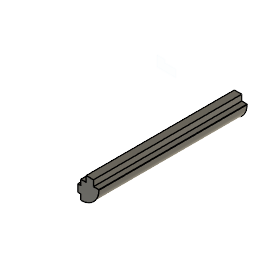
STOP LIGHT FINAL (Autodesk Fusion 360 archive; units mm, degrees)
design "FINAL STOP LIGHT CONNECTOR"
Autodesk Fusion 360 part; units mm, degrees
sketch "Sketch1" plane through (0, 0, 52.25) normal (0, 0, 1) x (-1, 0, 0)
  line L0 (12.25, -100) -> (12.25, 0)
  line L1 (12.25, 0) -> (0, 0)
  line L2 (0, 0) -> (0, -100)
  line L3 (0, -100) -> (12.25, -100)
  line L4 (0, 0) -> (12.25, 0) construction
  line L5 (6.125, 0) -> (8.625, 0) construction
  line L6 (6.125, 0) -> (3.625, 0) construction
  line L7 (3.625, 0) -> (8.625, 0) construction
  line L8 (3.625, 0) -> (8.625, 0)
  line L9 (8.625, 0) -> (8.625, -100)
  line L10 (8.625, -100) -> (3.625, -100)
  line L11 (3.625, -100) -> (3.625, 0)
  dimension "d3" = 5
  constraint coincident L1.end L2.start
  constraint coincident L0.end L1.start
  constraint midpoint L4 L5.start
  constraint horizontal L8
  constraint vertical L9
  constraint horizontal L10
  constraint vertical L11
  constraint coincident L3 L9.end
  measures "d3" distance of L6.end L5.end
sketch "Sketch2" plane through (0, 100, 0) normal (0, 1, 0) x (-1, 0, 0)
  line L0 (-4, 8.6) -> (-4, 3.6)
  line L1 (-4, 3.6) -> (8.5, 3.6)
  line L2 (8.5, 3.6) -> (8.5, 10.6)
  line L3 (8.5, 10.6) -> (3.5, 10.6)
  line L4 (3.5, 10.6) -> (3.5, 8.6)
  line L5 (3.5, 8.6) -> (-4, 8.6)
sketch "Sketch3" plane through (0, 100, 0) normal (0, 1, 0) x (-1, 0, 0)
  line L0 (-43.625, 52.25) -> (-43.625, 50.25)
  line L1 (-43.625, 50.25) -> (-48.625, 50.25)
  line L2 (-48.625, 50.25) -> (-48.625, 52.25)
  line L3 (-48.625, 52.25) -> (-52.25, 52.25)
  line L4 (-52.25, 52.25) -> (-52.25, 12.25)
  line L5 (-52.25, 12.25) -> (-48.625, 12.25)
  line L6 (-48.625, 12.25) -> (-48.625, 16.25)
  line L7 (-48.625, 16.25) -> (-43.625, 16.25)
  line L8 (-43.625, 16.25) -> (-43.625, 12.25)
  line L9 (-43.625, 12.25) -> (-40, 12.25)
  line L10 (-40, 12.25) -> (-40, 52.25)
  line L11 (-40, 52.25) -> (-43.625, 52.25)
  line L12 (-40, 0) -> (-56, 0) construction
  line L13 (-52.25, 12.25) -> (-48.625, 12.25)
  line L14 (-48.625, 16.25) -> (-48.625, 12.25)
  line L15 (-43.625, 16.25) -> (-48.625, 16.25)
  line L16 (-43.625, 12.25) -> (-43.625, 16.25)
  line L17 (-40, 12.25) -> (-43.625, 12.25)
  line L18 (-40, 8.6) -> (-40, 12.25)
  line L19 (-38, 8.6) -> (-40, 8.6)
  line L20 (-38, 3.6) -> (-38, 8.6)
  line L21 (-40, 3.6) -> (-38, 3.6)
  line L22 (-40, 0) -> (-40, 3.6)
  line L23 (-40, 0) -> (-52.25, 0)
  line L24 (-52.25, 12.25) -> (-52.25, 0)
  constraint coincident L4.end L5.start
  constraint horizontal L12
  constraint coincident L5.end L6.start
  constraint coincident L6.end L7.start
  constraint coincident L7.end L8.start
  constraint coincident L8.end L9.start
  constraint coincident L9.end L10.start
  constraint horizontal L19
  constraint perpendicular L19 L20
  constraint perpendicular L20 L21
  constraint coincident L12 L23.end
extrude "Extrude3" add sketch "Sketch3" against normal blind 100 contours L5 L6 L7 L8 L9 L13 L14 L15 L16 L17 L18 L19 L20 L21 L22 L23 L24
fillet "Fillet1" radius 12 1 edges at (52.25, 50, 0)

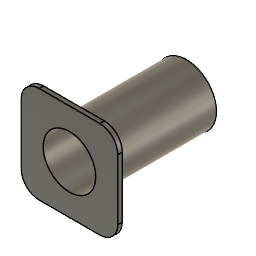
design "connector to base plate"
Autodesk Fusion 360 part; units mm, degrees
sketch "Sketch1" plane through (0, 0, 52.25) normal (0, 0, 1) x (-1, 0, 0)
  line L0 (12.25, -100) -> (12.25, 0)
  line L1 (12.25, 0) -> (0, 0)
  line L2 (0, 0) -> (0, -100)
  line L3 (0, -100) -> (12.25, -100)
  line L4 (0, 0) -> (12.25, 0) construction
  line L5 (6.125, 0) -> (8.625, 0) construction
  line L6 (6.125, 0) -> (3.625, 0) construction
  line L7 (3.625, 0) -> (8.625, 0) construction
  line L8 (3.625, 0) -> (8.625, 0)
  line L9 (8.625, 0) -> (8.625, -100)
  line L10 (8.625, -100) -> (3.625, -100)
  line L11 (3.625, -100) -> (3.625, 0)
  dimension "d3" = 5
  constraint coincident L1.end L2.start
  constraint coincident L0.end L1.start
  constraint midpoint L4 L5.start
  constraint horizontal L8
  constraint vertical L9
  constraint horizontal L10
  constraint vertical L11
  constraint coincident L3 L9.end
  measures "d3" distance of L6.end L5.end
extrude "Extrude1" add sketch "Sketch1" along normal blind 5 contours L1 L3 L8 L9 L10 L11
extrude "Extrude2" cut 1 faces at (-5.2917, 66.6667, 57.25) along direction (0, 0, -1) blind 10
sketch "Sketch2" plane through (0, 100, 0) normal (0, 1, 0) x (-1, 0, 0)
  line L0 (-4, 8.6) -> (-4, 3.6)
  line L1 (-4, 3.6) -> (8.5, 3.6)
  line L2 (8.5, 3.6) -> (8.5, 10.6)
  line L3 (8.5, 10.6) -> (3.5, 10.6)
  line L4 (3.5, 10.6) -> (3.5, 8.6)
  line L5 (3.5, 8.6) -> (-4, 8.6)
sketch "Sketch3" plane through (52.1964, 100, 12.1825) normal (0, 1, 0) x (0, 0, -1)
  line L0 (12.1825, 12.1964) -> (8.5825, 12.1964)
  line L1 (8.5825, 12.1964) -> (8.5825, 14.1964)
  line L2 (8.5825, 14.1964) -> (3.5825, 14.1964)
  line L3 (3.5825, 14.1964) -> (3.5825, 12.1964)
  line L4 (3.5825, 12.1964) -> (-0.0675, 12.1964)
  line L5 (-0.0675, 12.1964) -> (-0.0675, 8.5714)
  line L6 (-0.0675, 8.5714) -> (-4.0675, 8.5714)
  line L7 (-4.0675, 8.5714) -> (-4.0675, 3.5714)
  line L8 (-4.0675, 3.5714) -> (-0.0675, 3.5714)
  line L9 (-0.0675, 3.5714) -> (-0.0675, -0.0536)
  line L10 (-0.0675, -0.0536) -> (0.1825, -0.0536)
  line L11 (12.1825, 11.9464) -> (12.1825, 12.1964)
  line L12 (12.1825, 11.9464) -> (-52.2495, 11.9464)
  line L13 (-52.2495, 11.9464) -> (-52.2495, 76.3784)
  line L14 (-52.2495, 76.3784) -> (12.1825, 76.3784)
  line L15 (12.1825, 76.3784) -> (12.1825, 11.9464)
  arc A0 (0.1825, -0.0536) -> (12.1825, 11.9464) centre (0.1825, 11.9464) ccw
  dimension "d8" = 64.432
  dimension "d9" = 64.432
  constraint vertical L13
  constraint perpendicular L12 L13
  constraint horizontal L14
  constraint parallel L13 L15
  constraint coincident L11.start L12.start
  measures "d8" distance of L11.start L12.end
  measures "d9" distance of L11.start L14.end
extrude "Extrude3" add sketch "Sketch3" along normal blind 3 contours L0 L1 L2 L3 L4 L5 L11 L12 L15 | L0 L1 L2 L3 L4 L5 L12 L13 L14 L15
sketch "Sketch4" plane through (0, 103, 0) normal (0, 1, 0) x (-1, 0, 0)
  line L0 (24.182, 0) -> (24.182, 64.432)
  line L1 (24.182, 64.432) -> (-40.25, 64.432)
  line L2 (-40.25, 64.432) -> (-40.25, 0)
  line L3 (-40.25, 0) -> (24.182, 0)
  line L4 (24.182, 64.432) -> (-40.25, 0) construction
  line L5 (24.182, 0) -> (-40.25, 64.432) construction
  circle A0 centre (-8.034, 32.216) radius 17.5
  circle A1 centre (-8.034, 32.216) radius 20
  dimension "d12" = 35
  dimension "d13" = 40
  constraint coincident L0.end L1.start
  constraint coincident L2.end L3.start
  constraint coincident L0.start L3.end
  constraint coincident L1.end L2.start
  constraint midpoint L5 A0.centre
  constraint concentric A0 A1
  measures "d12" diameter of A0
  measures "d13" diameter of A1
extrude "Extrude4" add sketch "Sketch4" along normal blind 75 contours A1
extrude "Extrude5" cut 1 faces at (9.2669, 103, 37.0337) along direction (0, -1, 0) blind 16
move_body "Move1" bodies 1 to x (1, 0, 0) y (0, 1, 0) z (0, 0, 1) at (0, 0, -12)
sketch "Sketch5" plane through (0, 103, 0) normal (0, 1, 0) x (-1, 0, 0)
  line L0 (-40.25, -12) -> (24.182, -12)
  line L1 (24.182, -12) -> (24.182, 52.432)
  line L2 (24.182, 52.432) -> (-40.25, 52.432)
  line L3 (-40.25, 52.432) -> (-40.25, -12)
  circle A0 centre (-8.034, 20.216) radius 20
fillet "Fillet1" radius 12 4 edges at (40.25, 101.5, -12) (40.25, 101.5, 52.432) (-24.182, 101.5, 52.432) (-24.182, 101.5, -12)

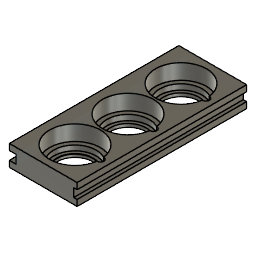
design "stop light"
Autodesk Fusion 360 part; units mm, degrees
sketch "Sketch1" plane through (0, 0, 0) normal (0, 0, 1) x (1, 0, 0)
  line L0 (0, 0) -> (40, 0)
  line L1 (40, 0) -> (40, 100)
  line L2 (40, 100) -> (0, 100)
  line L3 (0, 100) -> (0, 0)
  circle A0 centre (20, 50) radius 12.5
  circle A1 centre (20, 81.25) radius 12.5
  line L4 (5, 81.25, 3.25) -> (5, 66.25, 3.25)
  line L5 (5, 66.25, 3.25) -> (20, 66.25, 3.25)
  line L6 (35, 81.25, 3.25) -> (35, 96.25, 3.25)
  line L7 (35, 96.25, 3.25) -> (20, 96.25, 3.25)
  line L8 (35, 96.25, 3.25) -> (5, 96.25, 3.25)
  line L9 (5, 96.25, 3.25) -> (5, 66.25, 3.25)
  line L10 (5, 66.25, 3.25) -> (35, 66.25, 3.25)
  line L11 (35, 66.25, 3.25) -> (35, 96.25, 3.25)
  line L12 (5, 50, 3.25) -> (5, 65, 3.25)
  line L13 (5, 65, 3.25) -> (20, 65, 3.25)
  line L14 (35, 50, 3.25) -> (35, 35, 3.25)
  line L15 (35, 35, 3.25) -> (20, 35, 3.25)
  line L16 (35, 35, 3.25) -> (5, 35, 3.25)
  line L17 (5, 35, 3.25) -> (5, 65, 3.25)
  line L18 (5, 65, 3.25) -> (35, 65, 3.25)
  line L19 (35, 65, 3.25) -> (35, 35, 3.25)
  line L20 (5, 18.75, 3.25) -> (5, 3.75, 3.25)
  line L21 (5, 3.75, 3.25) -> (20, 3.75, 3.25)
  line L22 (35, 18.75, 3.25) -> (35, 33.75, 3.25)
  line L23 (35, 33.75, 3.25) -> (19.9836, 33.75, 3.25)
  line L24 (35, 33.75, 3.25) -> (5, 33.75, 3.25)
  line L25 (5, 33.75, 3.25) -> (5, 3.75, 3.25)
  line L26 (5, 3.75, 3.25) -> (35, 3.75, 3.25)
  line L27 (35, 3.75, 3.25) -> (35, 33.75, 3.25)
  circle A2 through (32.4836, 18.7208, 0.25) (13.7336, 29.5461, 0.25) (13.7336, 7.8955, 0.25)
  line L28 (5, 96.25, 3.25) -> (5, 100, 3.25) construction
  dimension "d1" = 40
  dimension "d2" = 100
  dimension "d11" = 25
  dimension "d15" = 25
  dimension "d55" = 25
  constraint horizontal L0
  constraint vertical L1
  constraint horizontal L2
  constraint vertical L3
  constraint coincident L0.start L3.end
  measures "d1" distance of L0.start L0.end
  measures "d2" distance of L0.start L2.end
  measures "d11" diameter of A0
  measures "d15" diameter of A1
extrude "Extrude1" add sketch "Sketch1" along normal blind 5 makes body 1
extrude "Extrude2" add sketch "Sketch1" against normal blind 2 separate body contours A0 | A1 makes body 2 at (19.2565, 46.7424, 0) makes body 3 at (19.0728, 79.6441, 0)
fillet "Fillet1" radius 2 4 faces at (19.0728, 79.6441, -2) (19.2565, 46.7424, -2) (19.2565, 46.7424, -2) (19.0728, 79.6441, -2) on bodies 2 3
extrude "Extrude3" cut 4 faces at (18.7213, 77.9918, -2) (17.2787, 53.4124, -2) (17.2787, 53.4124, -2) (18.7213, 77.9918, -2) along direction (0, 0, 1) blind 2 on bodies 2 3 bodies 2 3
extrude "Extrude7" cut sketch "Sketch1" along normal blind 10 contours L4 L5 L6 L7 L8 L9 L10 L11 | L12 L13 L14 L15 L16 L17 L18 L19 | L20 L21 L22 L23 L24 L25 L26 L27 in plane through (0, 0, 3.25) normal (0, 0, 1) bodies 1
extrude "Extrude8" add sketch "Sketch1" against normal blind 2 separate body contours A2 in plane through (0, 0, 0.25) normal (0, 0, 1) makes body 4
fillet "Fillet2" radius 2 1 faces at (16.5957, 18.0998, -1.75) on bodies 4
extrude "Extrude9" cut 1 faces at (23.1185, 23.5948, -1.75) along direction (0, 0, 1) blind 20 on bodies 4 bodies 1 4
extrude "Extrude10" cut 2 faces at (7.4992, 19.3439, 0.2497) (31.7315, 17.5781, 0.25) along direction (0, 0, 1) blind 8 on bodies 4 bodies 1
fillet "Fillet3" radius 15 4 edges at (5, 33.75, 4.125) (35, 33.75, 4.125) (5, 3.75, 4.125) (35, 3.75, 4.125) on bodies 1
fillet "Fillet4" radius 15 4 edges at (5, 65, 4.125) (35, 65, 4.125) (5, 35, 4.125) (35, 35, 4.125) on bodies 1
fillet "Fillet5" radius 15 4 edges at (5, 96.25, 4.125) (5, 66.25, 4.125) (35, 96.25, 4.125) (35, 66.25, 4.125) on bodies 1
extrude "Extrude11" add 1 faces at (1.6667, 49.999, 5) along direction (0, 0, 1) blind 7.25 on bodies 1 bodies 1
sketch "Sketch5" plane through (0, 0, 3.25) normal (0, 0, 1) x (1, 0, 0)
  line L0 (35, 81) -> (35, 85)
  circle A0 centre (35, 81) radius 2
  circle A1 centre (35, 50) radius 2
  circle A2 centre (35.0065, 18.7388) radius 2
  dimension "d85" = 4
  dimension "d86" = 4
  dimension "d87" = 4
  constraint vertical L0
  constraint coincident L0.start A0.centre
  measures "d85" diameter of A0
  measures "d86" diameter of A1
  measures "d87" diameter of A2
extrude "Extrude12" cut sketch "Sketch5" along normal blind 11 bodies 1
sketch "Sketch6" plane through (0, 0, 0) normal (-1, 0, 0) x (0, -1, 0)
  line L0 (-100, 0) -> (0, 0)
  line L1 (0, 0) -> (0, 12.25)
  line L2 (0, 12.25) -> (-100, 12.25)
  line L3 (-100, 12.25) -> (-100, 0)
  line L4 (0, 12.25) -> (0, 0) construction
  line L5 (0, 6.125) -> (0, 8.625) construction
  line L6 (0, 8.625) -> (-100, 8.625)
  line L7 (-100, 8.625) -> (-100, 3.625)
  line L8 (-100, 3.625) -> (0, 3.625)
  line L9 (0, 3.625) -> (0, 8.625)
  dimension "d90" = 2.5
  dimension "d91" = 100
  dimension "d92" = 5
  constraint coincident L1.end L2.start
  constraint coincident L0.end L1.start
  constraint midpoint L4 L5.start
  constraint perpendicular L0 L5
  constraint horizontal L6
  constraint vertical L7
  constraint horizontal L8
  constraint vertical L9
  measures "d90" distance of L5.start L5.end
  measures "d91" distance of L5.end L6.end
  measures "d92" distance of L5.end L8.end
extrude "Extrude13" cut sketch "Sketch6" against normal blind 4 contours L1 L3 L6 L7 L8 L9 bodies 1
sketch "Sketch7" plane through (4, 0, 0) normal (-1, 0, 0) x (0, -1, 0)
  line L0 (0, 3.625) -> (0, 8.625)
  line L1 (0, 8.625) -> (-100, 8.625)
  line L2 (-100, 8.625) -> (-100, 3.625)
  line L3 (-100, 3.625) -> (0, 3.625)
sketch "Sketch8" plane through (40, 0, 0) normal (1, 0, 0) x (0, 1, 0)
  line L0 (0, 0) -> (100, 0)
  line L1 (100, 0) -> (100, 12.25)
  line L2 (100, 12.25) -> (0, 12.25)
  line L3 (0, 12.25) -> (0, 0)
  line L4 (100, 6.125) -> (100, 8.625) construction
  line L5 (100, 8.625) -> (0, 8.625)
  line L6 (0, 8.625) -> (0, 3.625)
  line L7 (0, 3.625) -> (100, 3.625)
  line L8 (100, 3.625) -> (100, 8.625)
  dimension "d95" = 2.5
  dimension "d96" = 100
  dimension "d97" = 5
  constraint midpoint L1 L4.start
  constraint perpendicular L2 L4
  constraint horizontal L5
  constraint vertical L6
  constraint horizontal L7
  constraint vertical L8
  measures "d95" distance of L4.start L4.end
  measures "d96" distance of L4.end L5.end
  measures "d97" distance of L4.end L7.end
extrude "Extrude14" cut sketch "Sketch8" against normal blind 2 contours L1 L3 L5 L6 L7 L8 bodies 1
ref_plane "WorkPlane1" through (20, 18, 3) normal (0, 0, 1) x (1, 0, 0)
extrude "Extrude4" [rolled back] along distance 2 taper angle 0
extrude "Extrude5" [rolled back] along distance 3 taper angle 0
extrude "Extrude6" [rolled back] along distance 3 taper angle 0
